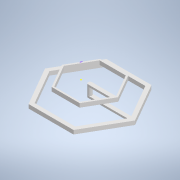
# Autodesk Inventor part: Part3
Saved by Autodesk Inventor 2020.2 (Build 242310000, 310)
## iProperties
Created: 2020-02-19
Part Number: Part3
Material: Generic
Document SubType Name: Modeling
Designer: lenovo
Density: 1 g/cm^3
Appearance: Default
Author: lenovo
Autodesk Inventor part; units mm, degrees
ref_plane "YZ Plane" through (0, 0, 0) normal (1, 0, 0) x (0, 1, 0)
ref_plane "XZ Plane" through (0, 0, 0) normal (0, 1, 0) x (-1, 0, 0)
ref_plane "XY Plane" through (0, 0, 0) normal (0, 0, 1) x (1, 0, 0)
sketch "Sketch1" plane through (0, 0, 0) normal (0, 1, 0) x (-1, 0, 0)
  line L0 (5.7735, 10) -> (11.547, 0)
  line L1 (11.547, 0) -> (5.7735, -10)
  line L2 (5.7735, -10) -> (-5.7735, -10)
  line L3 (-5.7735, -10) -> (-11.547, 0)
  line L4 (-11.547, 0) -> (-5.7735, 10)
  line L5 (-5.7735, 10) -> (5.7735, 10)
  line L6 (10.3923, 0) -> (5.1962, -9)
  line L7 (5.1962, -9) -> (-5.1962, -9)
  line L8 (-5.1962, -9) -> (-10.3923, 0)
  line L9 (-10.3923, 0) -> (-5.1962, 9)
  line L10 (-5.1962, 9) -> (5.1962, 9)
  line L11 (5.1962, 9) -> (10.3923, 0)
  line L12 (0, 0.5) -> (11.2583, 0.5)
  line L13 (0, 0) -> (5.7735, 10)
  line L14 (0, 0) -> (-5.7735, 10)
  line L15 (11.547, 0) -> (-11.547, 0)
  line L16 (0, 0.5) -> (-11.2583, 0.5)
  line L17 (-0.5, 0) -> (-6.0235, 9.567)
  line L18 (0.5, 0) -> (-5.2735, 10)
  line L19 (-0.5, 0) -> (5.2735, 10)
  line L20 (-0.5, 0) -> (11.047, 0) construction
  line L21 (0.5, 0) -> (6.0235, 9.567)
  line L22 (0, -0.5) -> (11.2583, -0.5)
  line L23 (0, 0) -> (5.7735, -10)
  line L24 (0, 0) -> (-5.7735, -10)
  line L25 (0, -0.5) -> (-11.2583, -0.5)
  line L26 (-0.5, 0) -> (-6.0235, -9.567)
  line L27 (0.5, 0) -> (-5.2735, -10)
  line L28 (-0.5, 0) -> (5.2735, -10)
  line L29 (0.5, 0) -> (6.0235, -9.567)
  point P0 (-10.1036, 0.5)
  point P1 (-5.4462, 8.567)
  point P2 (-0.7887, 0.5)
  point P3 (10.1036, 0.5)
  point P4 (0.7887, 0.5)
  point P5 (5.4462, 8.567)
  point P6 (4.6962, -9)
  point P7 (-4.6962, -9)
  point P8 (0, -0.866)
  point P9 (-5.4462, -8.567)
  point P10 (-10.1036, -0.5)
  point P11 (-0.7887, -0.5)
  point P12 (10.1036, -0.5)
  point P13 (5.4462, -8.567)
  point P14 (0.7887, -0.5)
  point P15 (-4.6962, 9)
  point P16 (4.6962, 9)
  point P17 (0, 0.866)
  dimension "d0" = 20
  dimension "d1" = 18
  dimension "d2" = 60
  constraints: 60 end point, 10 point on line, 7 symmetric about line, 2 coincident, 2 horizontal, 2 parallel, 1 equal length, 26 other
  measures "d0" distance between parallel lines of L2 L5
  measures "d1" distance between parallel lines of L7 L10
  measures "d2" angle of L20 L19
extrude "Extrusion1" add sketch "Sketch1" along normal blind 1 contours L13 L10 L19 L5 | L0 L21 L11 L13 | L0 L12 L11 L21 | L19 L10 L18 L5 | L13 L12 L18 L19 L10 | L11 L21 L12 L13 | L0 L15 L11 L12 | L18 L10 L14 L5 | L13 L18 L12 | L12 L21 L18 L13 | L1 L22 L6 L15 | L11 L15 L21 L12 | L14 L9 L17 L4 | L18 L19 L16 L14 L10 | L18 L12 L16 L19 | L18 L13 L14 L19 L16 L12 | L18 L15 L13 | L1 L29 L6 L22 | L6 L22 L29 L15 | L27 L23 L15 | L29 L22 L23 L27 | L17 L9 L16 L4 | L14 L16 L17 L9 | L19 L14 L16 | L15 L19 L14 | L24 L28 L15 | L23 L27 L22 L25 L28 L24 | L1 L23 L6 L29 | L23 L22 L27 | L29 L6 L23 L22 | L16 L9 L15 L4 | L14 L19 L17 L16 | L26 L25 L8 L15 | L15 L9 L16 L17 | L28 L24 L25 L26 | L28 L25 L24 | L2 L28 L7 L23 | L23 L7 L28 L27 L22 | L27 L28 L25 L22 | L15 L8 L25 L3 | L25 L24 L8 L26 | L25 L28 L27 L7 L24 | L2 L27 L7 L28 | L25 L8 L26 L3 | L8 L24 L3 L26 | L7 L27 L2 L24
sketch "Sketch2" plane through (0, 1, 0) normal (0, 1, 0) x (1, 0, 0)
  circle A0 centre (0, 0) radius 0.5
  dimension "d5" = 1
  constraints: 1 centre point, 1 coincident
  measures "d5" diameter of A0
extrude "Extrusion2" add sketch "Sketch2" along normal blind 2
sketch "Sketch3" plane through (0, 3, 0) normal (0, 1, 0) x (1, 0, 0)
  line L0 (-3.6084, -6.25) -> (-7.2169, 0)
  line L1 (-7.2169, 0) -> (-3.6084, 6.25)
  line L2 (-3.6084, 6.25) -> (3.6084, 6.25)
  line L3 (3.6084, 6.25) -> (7.2169, 0)
  line L4 (7.2169, 0) -> (3.6084, -6.25)
  line L5 (3.6084, -6.25) -> (-3.6084, -6.25)
  line L6 (-0.7887, -0.5) -> (-5.4462, -8.567) projected
  line L7 (-3.8584, -5.817) -> (3.1084, 6.25)
  line L8 (-5.4462, 8.567) -> (-0.7887, 0.5) projected
  line L9 (-3.8584, 5.817) -> (3.1084, -6.25)
  line L10 (-0.7887, 0.5) -> (-10.1036, 0.5) projected
  line L11 (-6.9282, 0.5) -> (6.9282, 0.5)
  line L12 (-10.1036, -0.5) -> (-0.7887, -0.5) projected
  line L13 (-6.9282, -0.5) -> (6.9282, -0.5)
  line L14 (0.7887, -0.5) -> (10.1036, -0.5) projected
  line L15 (-4.6962, -9) -> (0, -0.866) projected
  line L16 (-3.1084, -6.25) -> (3.8584, 5.817)
  line L17 (0, 0.866) -> (-4.6962, 9) projected
  line L18 (-3.1084, 6.25) -> (3.8584, -5.817)
  line L19 (-0.0006, -5.817) -> (3.8584, -5.817)
  line L20 (-0.0006, -5.817) -> (-3.8584, -5.817)
  line L21 (3.1084, -6.25) -> (6.9282, 0.5)
  line L22 (-3.1084, -6.25) -> (-6.9282, 0.5)
  line L23 (-7.2169, 0) -> (7.2169, 0)
  line L24 (-0.0006, 5.817) -> (3.8584, 5.817)
  line L25 (-0.0006, 5.817) -> (-3.8584, 5.817)
  line L26 (3.1084, 6.25) -> (6.9282, -0.5)
  line L27 (-3.1084, 6.25) -> (-6.9282, -0.5)
  point P0 (0, 0)
  point P1 (0, 0)
  point P2 (-2.8584, 5.817)
  point P3 (2.8584, 5.817)
  point P4 (-6.3623, 0.5)
  point P5 (-3.6034, 5.3753)
  point P6 (2.8584, -5.817)
  point P7 (-2.8584, -5.817)
  point P8 (-3.6034, -5.3753)
  point P9 (-6.3623, -0.5)
  point P10 (3.6034, -5.3753)
  point P11 (6.3623, -0.5)
  point P12 (6.3623, 0.5)
  point P13 (0.7887, 0.5)
  point P14 (3.6034, 5.3753)
  dimension "d8" = 12.5
  constraints: 42 end point, 19 point on line, 6 collinear, 1 coincident, 1 horizontal, 1 parallel, 1 symmetric about line, 13 other
  measures "d8" distance between parallel lines of L2 L5
extrude "Extrusion3" add sketch "Sketch3" along normal blind 1 contours L0 L20 L22 L5 | L0 L12 L22 L6 | L6 L22 L20 | L15 L20 L19 L9 L5 | L22 L20 L15 | L27 L22 L12 | L0 L23 L27 | L6 L13 L9 L15 L20 L22 | L21 L19 L4 L5 | L9 L19 L21 | L1 L22 L23 | L22 L23 L7 L12 | L27 L10 L9 L23 | L22 L10 L27 | L7 L9 L13 | L9 L16 L13 L18 L21 L19 | L21 L18 L19 | L9 L13 L16 | L1 L8 L27 L10 | L9 L11 L7 | L23 L16 L13 L9 | L7 L11 L18 L23 | L18 L21 L13 L4 | L16 L18 L13 | L25 L27 L8 | L1 L2 L27 L25 | L11 L8 L27 L25 L17 L7 | L7 L18 L11 | L18 L11 L16 | L23 L21 L13 L18 | L16 L11 L26 L23 | L26 L23 L4 | L13 L21 L26 | L27 L17 L25 | L7 L24 L26 L16 L11 L18 | L26 L11 L21 | L21 L3 L23 | L2 L7 L24 L25 L17 | L7 L26 L24 | L26 L16 L3 L11 | L26 L24 L16 | L2 L3 L24 L26
sketch "Sketch4" plane through (0, 4, 0) normal (0, 1, 0) x (1, 0, 0)
  line L0 (-2.8584, 5.817) -> (2.8584, 5.817) projected
  line L1 (3.3584, 5.817) -> (6.7169, 0)
  line L2 (6.7169, 0) -> (3.3584, -5.817)
  line L3 (3.3584, -5.817) -> (-3.3584, -5.817)
  line L4 (-3.3584, -5.817) -> (-6.7169, 0)
  line L5 (-6.7169, 0) -> (-3.3584, 5.817)
  line L6 (-3.3584, 5.817) -> (3.3584, 5.817)
  circle A0 centre (0, 0) radius 0.5 projected
  line L7 (0, 0.5) -> (6.4282, 0.5)
  line L8 (6.4282, -0.5) -> (0, -0.5)
  arc A1 (0, 0.5) -> (0, -0.5) centre (0, 0) ccw
  point P0 (0, 5.817)
  constraints: 16 end point, 5 point on circle, 4 tangent, 2 midpoint, 2 point on line, 1 centre point, 1 coincident, 1 horizontal, 13 other
extrude "Extrusion4" cut sketch "Sketch4" against normal blind 1 contours L0 L6 L1 L7 A0 L8 L2 L3 L4 L5
sketch "Sketch5" plane through (0, 4, 0) normal (0, 1, 0) x (1, 0, 0)
  line L0 (3.3584, 5.817) -> (6.4282, 0.5) projected
  line L1 (6.2201, 0.8605) -> (6.7169, 0)
  line L2 (0, -0.5) -> (6.4282, -0.5) projected
  line L3 (6.7169, 0) -> (6.4282, -0.5)
  line L4 (6.4282, -0.5) -> (0, -0.5)
  circle A0 centre (0, 0) radius 0.5 projected
  arc A1 (0, 0.5) -> (0, -0.5) centre (0, 0) ccw
  line L5 (0, 0.5) -> (6.2201, 0.8605)
  constraints: 8 end point, 3 point on circle, 2 collinear, 1 centre point, 1 point on line, 1 tangent
extrude "Extrusion5" cut sketch "Sketch5" against normal blind 0.5
sketch "Sketch6" plane through (0, 0, 0) normal (0, -1, 0) x (1, 0, 0)
  line L0 (10.3923, 0) -> (5.1962, -9)
  line L1 (5.1962, -9) -> (-5.1962, -9)
  line L2 (-5.1962, -9) -> (-10.3923, 0)
  line L3 (-10.3923, 0) -> (-5.1962, 9)
  line L4 (-5.1962, 9) -> (5.1962, 9)
  line L5 (5.1962, 9) -> (10.3923, 0)
  line L6 (10.1036, -0.5) -> (0, -0.5)
  line L7 (0.7887, 0.5) -> (10.1036, 0.5) projected
  line L8 (6.4282, 0.5) -> (0, 0.5) projected
  line L9 (0, -0.5) -> (0, 0.5)
  line L10 (0, 0.5) -> (10.1036, 0.5)
  arc A0 (0, 0.5) -> (0, -0.5) centre (0, 0) ccw projected
  arc A1 (0, 0.5) -> (0, -0.5) centre (0, 0) ccw
  dimension "d15" = 18
  constraints: 18 end point, 2 perpendicular, 2 point on circle, 2 point on line, 1 centre point, 1 coincident, 1 parallel, 1 tangent, 13 other
  measures "d15" distance between parallel lines of L1 L4
extrude "Extrusion6" cut sketch "Sketch6" against normal blind 1 contours L0 L1 L2 L3 L4 L5 L7 L8 A0 L6
sketch "Sketch7" plane through (0, 0, 0) normal (0, -1, 0) x (1, 0, 0)
  line L0 (10.1036, 0.5) -> (5.1962, 9) projected
  line L1 (9.7836, 1.0542) -> (10.3923, 0)
  line L2 (10.3923, 0) -> (10.1036, -0.5)
  line L3 (10.1036, -0.5) -> (0, -0.5)
  arc A0 (0, 0.5) -> (0, -0.5) centre (0, 0) ccw
  line L4 (0, 0.5) -> (9.7836, 1.0542)
  point P0 (0, 0)
  constraints: 8 end point, 2 point on circle, 1 centre point, 1 collinear, 1 horizontal, 1 point on line, 1 tangent
extrude "Extrusion7" cut sketch "Sketch7" against normal blind 0.5
sketch "Sketch8" plane through (-7.2169, 3, 0) normal (-0.866, 0, -0.5) x (-0.5, 0, 0.866)
  line L0 (-4.0415, 0.5) -> (-3.1084, 0.5) projected
  circle A0 centre (-3.6084, 0.5) radius 0.5022
  point P0 (-3.6084, -3)
  point P1 (-3.1754, 0.5)
  constraints: 1 centre point, 1 point on line
body "Solid1"
